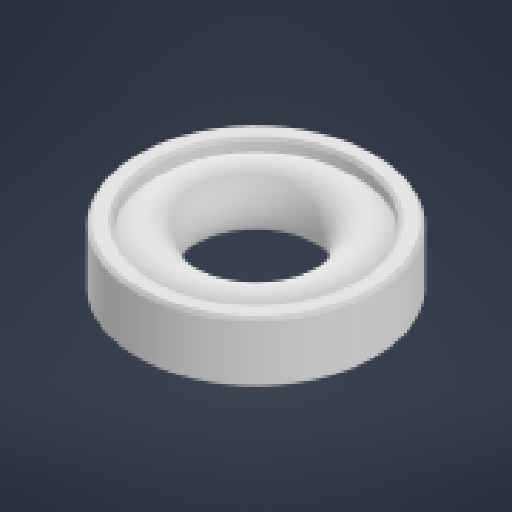
# Autodesk Inventor part: Outer_Ring
Saved by Autodesk Inventor 2023 (Build 270158000, 158)
## iProperties
Created: 2023-02-24
Part Number: Outer_Ring
Material: Generic
Document SubType Name: Modeling
Designer: izack
Density: 1 g/cm^3
Appearance: Default
Author: izack
Autodesk Inventor part; units mm, degrees
ref_plane "YZ Plane" through (0, 0, 0) normal (1, 0, 0) x (0, 1, 0)
ref_plane "XZ Plane" through (0, 0, 0) normal (0, 1, 0) x (-1, 0, 0)
ref_plane "XY Plane" through (0, 0, 0) normal (0, 0, 1) x (1, 0, 0)
sketch "Sketch1" plane through (0, 0, 0) normal (0, 0, 1) x (1, 0, 0)
  line L0 (9.5781, 5.4762) -> (1.5781, 5.4762) construction
  line L1 (9.5781, 0.4762) -> (1.5781, 0.4762) construction
  line L2 (13.8281, 0.4762) -> (15.3281, 0.4762)
  line L3 (15.3281, 0.4762) -> (15.3281, 5.4762)
  line L4 (15.3281, 5.4762) -> (13.8281, 5.4762)
  line L5 (13.8281, 5.4762) -> (13.8281, 0.4762)
  line L6 (5.5781, 5.4762) -> (5.5781, 0.4762) construction
  line L7 (15.3281, 2.9762) -> (5.5781, 2.9762) construction
  circle A0 centre (12.0781, 2.9762) radius 2.25
  point P0 (0, 0)
  point P1 (13.8281, 4.3904)
  point P2 (13.8281, 1.562)
  point P3 (3.0119, 0.4762)
  dimension "d1" = 5
  dimension "d2" = 19.5
  dimension "d3" = 4.5
  dimension "d4" = 1.75
  dimension "d5" = 1.5
  constraints: 12 end point, 4 midpoint, 2 parallel, 2 point on line, 1 centre point, 1 horizontal, 1 perpendicular
  measures "d1" distance of L2.end L3.end
  measures "d2" diameter of L3 L6
  measures "d3" diameter of A0
  measures "d4" distance from line of L5 A0.centre
  measures "d5" distance between parallel lines of L3 L5
revolve "Revolution1" add sketch "Sketch1" angle 360 about axis through (5.5781, 5.4762, 0) along (0, -1, 0) contours L5 A0 L4 L3 L2
chamfer "Chamfer1" distance 0.25 angle 45 4 edges at (-4.1719, 5.4762, 0) (-2.6719, 5.4762, 0) (-4.1719, 0.4762, 0) (-2.6719, 0.4762, 0)
equation "\"d2\" = do"
equation "\"do\" = 19.5"
body "Solid1"
